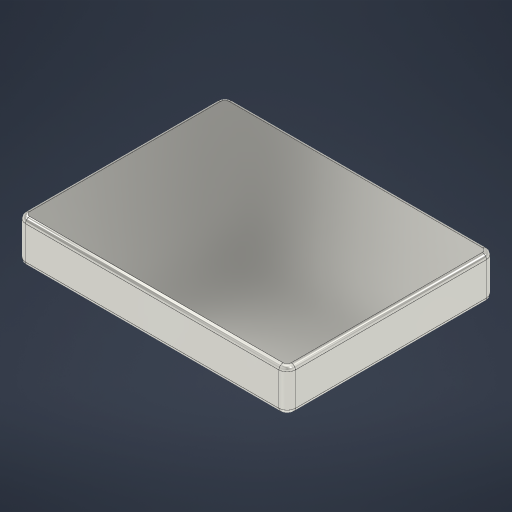
# Autodesk Inventor part: battery_surrogate
Saved by Autodesk Inventor 2024.2 (Build 282272000, 272)
## iProperties
Created: 2025-05-21
Part Number: battery_surrogate
Material: Generic
Document SubType Name: Modeling
Designer: Moe
Density: 1 g/cm^3
Appearance: Default
Author: Moe
Autodesk Inventor part; units mm, degrees
ref_plane "YZ Plane" through (0, 0, 0) normal (1, 0, 0) x (0, 1, 0)
ref_plane "XZ Plane" through (0, 0, 0) normal (0, 1, 0) x (-1, 0, 0)
ref_plane "XY Plane" through (0, 0, 0) normal (0, 0, 1) x (1, 0, 0)
sketch "Sketch1" plane through (0, 0, 0) normal (0, 1, 0) x (-1, 0, 0)
  line L0 (1, 0) -> (31.5, 0)
  line L1 (32.5, -1) -> (32.5, -24)
  line L2 (31.5, -25) -> (1, -25)
  line L3 (0, -24) -> (0, -1)
  arc A0 (32.5, -1) -> (31.5, 0) centre (31.5, -1) ccw
  arc A1 (31.5, -25) -> (32.5, -24) centre (31.5, -24) ccw
  arc A2 (1, 0) -> (0, -1) centre (1, -1) ccw
  arc A3 (0, -24) -> (1, -25) centre (1, -24) ccw
  point P0 (0, 0)
  point P1 (32.5, -25)
  point P2 (32.5, 0)
  point P3 (0, -25)
  dimension "d0" = 32.5
  dimension "d1" = 25
  dimension "d2" = 1
  constraints: 8 end point, 8 point on circle, 8 point on line, 8 tangent, 4 centre point, 3 equal radius, 2 parallel, 1 horizontal, 1 perpendicular
  measures "d0" distance of point (32.5, -25) point (0, -25)
  measures "d1" distance of point (32.5, 0) point (32.5, -25)
  measures "d2" radius of A0
extrude "Extrusion1" add sketch "Sketch1" along normal blind 5
fillet "Fillet1" radius 0.5 16 edges at (-16.25, 0, -25) (-32.2071, 0, -24.7071) (-32.5, 0, -12.5) (-32.2071, 0, -0.2929) (-16.25, 0, 0) (-0.2929, 0, -0.2929) (0, 0, -12.5) (-0.2929, 0, -24.7071) (-16.25, 5, -25) (-32.2071, 5, -24.7071) (-32.5, 5, -12.5) (-32.2071, 5, -0.2929) (-16.25, 5, 0) (-0.2929, 5, -0.2929) (0, 5, -12.5) (-0.2929, 5, -24.7071)
body "Solid1"
